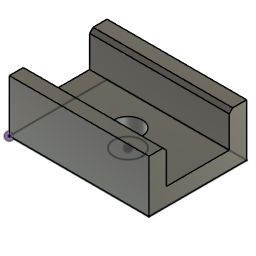
Dowel Template 18mm (Autodesk Fusion 360 design; units mm, degrees)
Autodesk Fusion 360 part; units mm, degrees
sketch "Sketch1" plane through (0, 0, 0) normal (0, 0, 1) x (1, 0, 0)
  line L0 (0, 0) -> (40, 0)
  line L1 (40, 0) -> (40, 28)
  line L2 (40, 28) -> (0, 28)
  line L3 (0, 28) -> (0, 0)
  circle A0 centre (20, 14) radius 4.05
  dimension "d1" = 40
  dimension "d2" = 28
  dimension "d3" = 8.1
  dimension "d10" = 14
  dimension "d11" = 20
  constraint horizontal L0
  constraint vertical L1
  constraint horizontal L2
  constraint vertical L3
  constraint coincident L0.start L3.end
  measures "d1" distance of L0.start L0.end
  measures "d2" distance of L0.start L2.end
  measures "d3" diameter of A0
  measures "d10" distance of L0 A0.centre
  measures "d11" distance of L1 A0.centre
extrude "Extrude1" add sketch "Sketch1" along normal blind 5
sketch "Sketch2" plane through (0, 0, 5) normal (0, 0, 1) x (-1, 0, 0)
  circle A0 centre (-20, -14) radius 4.05
  line L0 (0, -28) -> (0, 0)
  line L1 (0, 0) -> (-40, 0)
  line L2 (-40, 0) -> (-40, -28)
  line L3 (-40, -28) -> (0, -28)
  line L4 (0, -28) -> (-40, -28)
  line L5 (-40, -28) -> (-40, -23)
  line L6 (-40, -23) -> (0, -23)
  line L7 (0, -23) -> (0, -28)
  line L8 (0, 0) -> (-40, 0)
  line L9 (-40, 0) -> (-40, -5)
  line L10 (-40, -5) -> (0, -5)
  line L11 (0, -5) -> (0, 0)
  dimension "d6" = 40
  dimension "d7" = 5
  dimension "d8" = 40
  dimension "d9" = 5
  constraint horizontal L4
  constraint vertical L5
  constraint horizontal L6
  constraint vertical L7
  constraint coincident L0.start L3.end
  constraint horizontal L8
  constraint vertical L9
  constraint horizontal L10
  constraint vertical L11
  constraint coincident L0.end L1.start
  measures "d6" distance of L0.start L2.end
  measures "d7" distance of L0.start L6.end
  measures "d8" distance of L0.end L1.end
  measures "d9" distance of L0.end L10.end
extrude "Extrude2" add sketch "Sketch2" along normal blind 10 contours L0 L2 L3 L4 L5 L6 L7 | L0 L1 L2 L8 L9 L10 L11
chamfer "Chamfer1" distance 1 angle 45 2 edges at (20, 23, 15) (20, 5, 15)
sketch "Sketch3" plane through (0, 0, 0) normal (0, 0, 1) x (1, 0, 0)
  circle A0 centre (20, 14) radius 6
  circle A1 centre (20, 14) radius 4.05
  dimension "d15" = 12
  measures "d15" diameter of A0
extrude "Extrude3" add sketch "Sketch3" against normal blind 5
